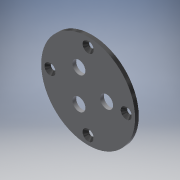
# Autodesk Inventor part: anschluss_daten
Saved by Autodesk Inventor 2018 (Build 220112000, 112)
## iProperties
Created: 2019-02-21
Part Number: anschluss_daten
Material: Generisch
Document SubType Name: Modeling
Designer: das RoboSAx OrgaTeam (pw)
Density: 1 g/cm^3
Appearance: Vorgabe
Project: RoboSAX Spielfeld
Author: das RoboSAx OrgaTeam (pw)
Autodesk Inventor part; units mm, degrees
ref_plane "YZ Plane" through (0, 0, 0) normal (1, 0, 0) x (0, 1, 0)
ref_plane "XZ Plane" through (0, 0, 0) normal (0, 1, 0) x (-1, 0, 0)
ref_plane "XY Plane" through (0, 0, 0) normal (0, 0, 1) x (1, 0, 0)
sketch "Skizze1" plane through (0, 0, 0) normal (0, 1, 0) x (-1, 0, 0)
  circle A0 centre (0, 0) radius 25.4
  dimension "d0" = 50.8
  constraints: 1 centre point, 1 coincident
  measures "d0" diameter of A0
extrude "Extrusion1" add sketch "Skizze1" along normal blind 2
sketch "Skizze2" plane through (0, 0, 0) normal (0, -1, 0) x (1, 0, 0)
  circle A0 centre (0, 0) radius 25.4 projected
  line L0 (-20.6475, 0) -> (0, 20.6475) construction
  line L1 (0, 20.6475) -> (20.6475, 0) construction
  line L2 (20.6475, 0) -> (0, -20.6475) construction
  line L3 (0, -20.6475) -> (-20.6475, 0) construction
  line L4 (0, 0) -> (10.3238, 10.3238) construction
  line L5 (0, 0) -> (-10.3238, 10.3238) construction
  circle A1 centre (0, 0) radius 25.4 construction
  line L6 (0, 0) -> (0, 25.4) construction
  point P0 (-20.6475, 0)
  point P1 (0, 20.6475)
  point P2 (20.6475, 0)
  dimension "d3" = 29.2
  dimension "d4" = 29.2
  dimension "d63" = 45
  constraints: 14 end point, 4 coincident, 3 perpendicular, 2 midpoint, 2 parallel, 1 vertical, 1 vertical alignment, 1 other
  measures "d3" distance of L0.start L0.end
  measures "d4" distance of L0.end L1.end
  measures "d63" angle of L6 L5
hole "Bohrung1" at (-20.6475, 0, 0) at (0, 0, 20.6475) at (20.6475, 0, 0) at (0, 0, -20.6475) direction (0, 1, 0) diameter 3 end through all countersink diameter 6 countersink angle 90
sketch "Skizze7" plane through (0, 0, 0) normal (0, -1, 0) x (1, 0, 0)
  circle A0 centre (0, 0) radius 25.4 construction
  circle A1 centre (0, 0) radius 10 construction
  line L0 (0, 0) -> (10, 0) construction
  circle A2 centre (0, 0) radius 10 construction
  line L1 (0, 0) -> (-5, 8.6603) construction
  circle A3 centre (0, 0) radius 10 construction
  line L2 (0, 0) -> (-5, -8.6603) construction
  dimension "d68" = 20
  dimension "d71" = 360
  constraints: 6 end point, 4 coincident, 1 horizontal, 1 horizontal alignment, 22 other
hole "Bohrung3" at (-5, 0, 8.6603) at (10, 0, 0) at (-5, 0, -8.6603) direction (0, 1, 0) diameter 7 end through all
